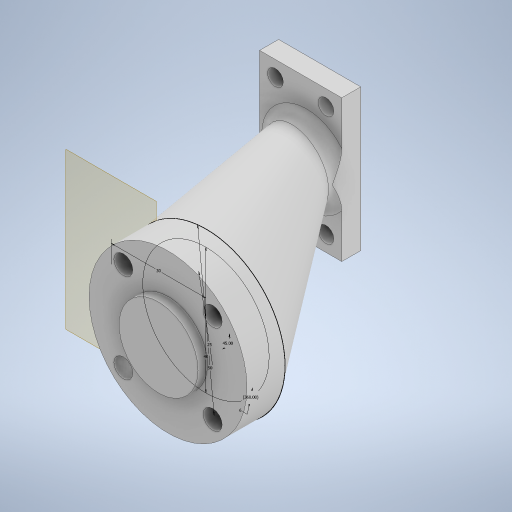
# Autodesk Inventor part: conexión
Saved by Autodesk Inventor 2024.3 (Build 283343000, 343)
## iProperties
Created: 2025-07-08
Part Number: conexión
Material: Generic
Document SubType Name: Modeling
Designer: user
Density: 1 g/cm^3
Appearance: Default
Author: user
Autodesk Inventor part; units mm, degrees
ref_plane "YZ Plane" through (0, 0, 0) normal (1, 0, 0) x (0, 1, 0)
ref_plane "XZ Plane" through (0, 0, 0) normal (0, 1, 0) x (-1, 0, 0)
ref_plane "XY Plane" through (0, 0, 0) normal (0, 0, 1) x (1, 0, 0)
sketch "Sketch1" plane through (0, 0, 0) normal (0, 0, 1) x (1, 0, 0)
  line L0 (-13, 22.45) -> (13, 22.45) projected
  line L1 (-13, -22.45) -> (-13, 22.45) projected
  line L2 (13, -22.45) -> (-13, -22.45) projected
  line L3 (13, 22.45) -> (13, -22.45) projected
  line L4 (0, 0) -> (8, 0)
  line L5 (8, 0) -> (8, -17.5)
  circle A0 centre (8, -17.5) radius 2.5
  circle A1 centre (-19.1601, -1.7726) radius 2.5
  line L6 (0, -22.45) -> (0, 22.45)
  circle A2 centre (-8, -17.5) radius 2.5
  line L7 (13, 0) -> (-13, 0)
  circle A3 centre (8, 17.5) radius 2.5
  circle A4 centre (-8, 17.5) radius 2.5
  circle A5 centre (8, -17.5) radius 2.5 projected
  circle A6 centre (-8, 17.5) radius 2.5 projected
  circle A7 centre (-8, -17.5) radius 2.5 projected
  circle A8 centre (8, 17.5) radius 2.5 projected
  dimension "d1" = 8
  dimension "d2" = 17.5
  dimension "d3" = 5
  constraints: 8 end point, 5 centre point, 4 midpoint, 3 symmetric about line, 1 coincident, 1 horizontal, 1 perpendicular, 3 other
  measures "d1" distance of L4.start L4.end
  measures "d2" distance of L4.end L5.end
  measures "d3" diameter of A0
extrude "Extrusion1" add sketch "Sketch1" along normal blind 6 contours L0 L6 L7 L1 | L0 L3 L7 L4 L6 | L7 L6 L2 L1 | L4 L7 L3 L2 L6
sketch "Sketch2" plane through (0, 0, 6) normal (0, 0, 1) x (1, 0, 0)
  circle A0 centre (0, 0) radius 10
  dimension "d6" = 20
  constraints: 1 centre point, 1 coincident
  measures "d6" diameter of A0
ref_plane "Work Plane1" through (0, 0, 66) normal (0, 0, 1) x (1, 0, 0)
sketch "Sketch3" plane through (0, 0, 66) normal (0, 0, 1) x (1, 0, 0)
  line L0 (0, 0) -> (30, 0)
  circle A0 centre (30, 0) radius 25
  circle A1 centre (30, 0) radius 20
  line L1 (30, 0) -> (47.6777, -17.6777)
  line L2 (30, 0) -> (55, 0) construction
  circle A2 centre (44.1421, -14.1421) radius 3
  circle A3 centre (44.1421, 14.1421) radius 3
  circle A4 centre (15.8579, 14.1421) radius 3
  circle A5 centre (15.8579, -14.1421) radius 3
  circle A6 centre (30, 0) radius 12.5
  dimension "d10" = 50
  dimension "d11" = 40
  dimension "d8" = 30
  dimension "d12" = 45
  dimension "d13" = 6
  dimension "d16" = 360
  dimension "d18" = 25
  constraints: 6 end point, 5 centre point, 4 coincident, 2 horizontal, 1 equal length, 1 point on line, 15 other
  measures "d8" distance of L0.start L0.end
  measures "d12" angle of L1 L2
  measures "d13" diameter of A2
  measures "d18" diameter of A6
extrude "Extrusion2" add sketch "Sketch3" along normal blind 12 contours A0 L1 A2 A1 A3 A4 L0 | L0 A1 A5 A2 L1 A0 | A1 A4 A3 A2 L1 A6 L0 | L0 A6 L1 A2 A1 A5
extrude "Extrusion3" add sketch "Sketch3" along normal blind 15 contours A6 L1 L0 | L0 L1 A6
loft "Loft1" add profiles "Sketch2", "Sketch3"
fillet "Fillet1" radius 3 1 edges at (-10, 0, 6)
body "Solid1"
